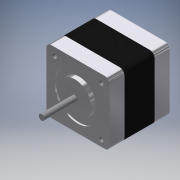
# Autodesk Inventor part: Nema17 - 40mm BRUG DENNE
Saved by Autodesk Inventor 2016 SP1 (Build 200210100, 210)
## iProperties
Created: 2012-03-17
Part Number: Nema17 - 40mm BRUG DENNE
Material: Generic
Document SubType Name: Modeling
Designer: Matt
Density: 1 g/cm^3
Appearance: Default
Author: Matt
Autodesk Inventor part; units mm, degrees
ref_plane "YZ Plane" through (0, 0, 0) normal (1, 0, 0) x (0, 1, 0)
ref_plane "XZ Plane" through (0, 0, 0) normal (0, 1, 0) x (-1, 0, 0)
ref_plane "XY Plane" through (0, 0, 0) normal (0, 0, 1) x (1, 0, 0)
sketch "Sketch1" plane through (0, 0, 0) normal (0, 0, 1) x (1, 0, 0)
  line L0 (-7.9846, 3.5499) -> (34.0154, 3.5499)
  line L1 (34.0154, 3.5499) -> (34.0154, -38.4501)
  line L2 (34.0154, -38.4501) -> (-7.9846, -38.4501)
  line L3 (-7.9846, -38.4501) -> (-7.9846, 3.5499)
  circle A0 centre (12.8654, -17.3001) radius 11
  circle A1 centre (12.8654, -17.3001) radius 1.891
  circle A2 centre (12.8654, -17.3001) radius 15.5
  circle A3 centre (-2.6346, -32.8001) radius 1.5
  circle A4 centre (28.3654, -34.3001) radius 1.5
  circle A5 centre (28.3654, -1.8001) radius 1.5
  circle A6 centre (-2.6346, -1.8001) radius 1.5
  point P0 (0, 0)
  dimension "d0" = 42
  dimension "d1" = 42
  dimension "d2" = 22
  dimension "d3" = 31
  dimension "d4" = 3
  dimension "d5" = 3
  dimension "d6" = 3
  dimension "d7" = 3
  constraints: 8 end point, 7 centre point, 2 coincident, 2 parallel, 1 horizontal, 1 perpendicular
  measures "d0" distance of L1.end L2.end
  measures "d1" distance of L0.end L1.end
  measures "d2" diameter of A0
  measures "d3" diameter of A2
  measures "d4" diameter of A3
  measures "d5" diameter of A4
  measures "d6" diameter of A5
  measures "d7" diameter of A6
extrude "Extrusion1" add sketch "Sketch1" along normal blind 40 contours L0 L1 L2 L3 | A0 | A1 | A2
fillet "Fillet1" radius 3.175 4 edges at (34.0154, 3.5499, 20) (-7.9846, 3.5499, 20) (34.0154, -38.4501, 20) (-7.9846, -38.4501, 20)
sketch "Sketch2" plane through (0, 0, 40) normal (0, 0, 1) x (1, 0, 0)
  circle A0 centre (12.8654, -17.3001) radius 15.5 projected
  circle A1 centre (12.8654, -17.3001) radius 1.891 projected
  circle A2 centre (12.8654, -17.3001) radius 11 projected
  point P0 (0, 0)
extrude "Extrusion2" add sketch "Sketch2" along normal blind 2 contours A2
sketch "Sketch3" plane through (0, 0, 40) normal (0, 0, 1) x (1, 0, 0)
  circle A0 centre (12.8654, -17.3001) radius 11 projected
  circle A1 centre (12.8654, -17.3001) radius 15.5 projected
  point P0 (0, 0)
extrude "Extrusion3" cut sketch "Sketch3" against normal blind 1
sketch "Sketch4" plane through (12.8654, -17.3001, 42) normal (0, 0, 1) x (1, 0, 0)
  circle A0 centre (0, 0) radius 1.891 projected
  point P0 (-12.8654, 17.3001)
extrude "Akse længde" add sketch "Sketch4" along normal blind 22
sketch "Sketch5" plane through (0, 0, 40) normal (0, 0, 1) x (1, 0, 0)
  arc A0 (-7.9846, -35.2751) -> (-4.8096, -38.4501) centre (-4.8096, -35.2751) ccw projected
  line L0 (30.8404, -38.4501) -> (-4.8096, -38.4501) projected
  arc A1 (30.8404, -38.4501) -> (34.0154, -35.2751) centre (30.8404, -35.2751) ccw projected
  line L1 (34.0154, 0.3749) -> (34.0154, -35.2751) projected
  arc A2 (34.0154, 0.3749) -> (30.8404, 3.5499) centre (30.8404, 0.3749) ccw projected
  line L2 (-4.8096, 3.5499) -> (30.8404, 3.5499) projected
  arc A3 (-4.8096, 3.5499) -> (-7.9846, 0.3749) centre (-4.8096, 0.3749) ccw projected
  line L3 (-7.9846, -35.2751) -> (-7.9846, 0.3749) projected
  arc A4 (34.0254, 0.3749) -> (30.8404, 3.5599) centre (30.8404, 0.3749) ccw
  line L4 (34.0254, 0.3749) -> (34.0254, -35.2751)
  arc A5 (30.8404, -38.4601) -> (34.0254, -35.2751) centre (30.8404, -35.2751) ccw
  line L5 (30.8404, -38.4601) -> (-4.8096, -38.4601)
  arc A6 (-7.9946, -35.2751) -> (-4.8096, -38.4601) centre (-4.8096, -35.2751) ccw
  line L6 (-7.9946, -35.2751) -> (-7.9946, 0.3749)
  arc A7 (-4.8096, 3.5599) -> (-7.9946, 0.3749) centre (-4.8096, 0.3749) ccw
  line L7 (-4.8096, 3.5599) -> (30.8404, 3.5599)
  point P0 (0, 0)
  dimension "d21" = 0.01
  constraints: 8 end point, 8 point on circle, 4 centre point, 7 other
  measures "d21" distance between parallel lines of L3 L6
extrude "Extrusion5" add sketch "Sketch5" against normal blind 10
sketch "Sketch6" plane through (0, 0, 0) normal (0, 0, -1) x (-1, 0, 0)
  arc A0 (4.8096, -38.4501) -> (7.9846, -35.2751) centre (4.8096, -35.2751) ccw projected
  line L0 (7.9846, -35.2751) -> (7.9846, 0.3749) projected
  arc A1 (7.9846, 0.3749) -> (4.8096, 3.5499) centre (4.8096, 0.3749) ccw projected
  line L1 (4.8096, 3.5499) -> (-30.8404, 3.5499) projected
  arc A2 (-30.8404, 3.5499) -> (-34.0154, 0.3749) centre (-30.8404, 0.3749) ccw projected
  line L2 (-34.0154, 0.3749) -> (-34.0154, -35.2751) projected
  arc A3 (-34.0154, -35.2751) -> (-30.8404, -38.4501) centre (-30.8404, -35.2751) ccw projected
  line L3 (-30.8404, -38.4501) -> (4.8096, -38.4501) projected
  line L4 (7.9946, 0.3749) -> (7.9946, -35.2751)
  arc A4 (4.8096, -38.4601) -> (7.9946, -35.2751) centre (4.8096, -35.2751) ccw
  line L5 (4.8096, -38.4601) -> (-30.8404, -38.4601)
  arc A5 (-34.0254, -35.2751) -> (-30.8404, -38.4601) centre (-30.8404, -35.2751) ccw
  line L6 (-34.0254, -35.2751) -> (-34.0254, 0.3749)
  arc A6 (-30.8404, 3.5599) -> (-34.0254, 0.3749) centre (-30.8404, 0.3749) ccw
  line L7 (-30.8404, 3.5599) -> (4.8096, 3.5599)
  arc A7 (7.9946, 0.3749) -> (4.8096, 3.5599) centre (4.8096, 0.3749) ccw
  point P0 (0, 0)
  dimension "d22" = 0.01
  constraints: 8 end point, 8 point on circle, 4 centre point, 7 other
  measures "d22" distance between parallel lines of L4 L0
extrude "Extrusion6" add sketch "Sketch6" against normal blind 10
body "Solid1"
